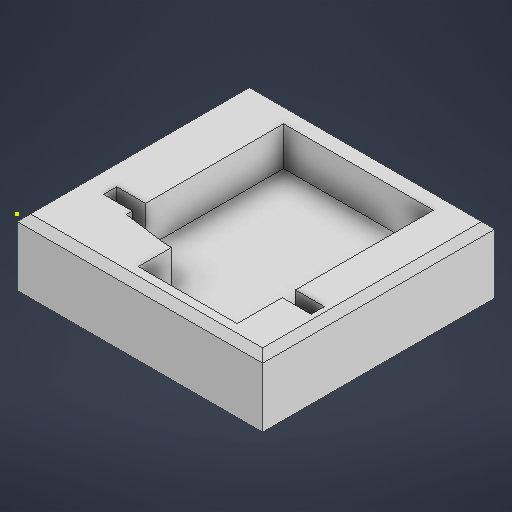
# Autodesk Inventor part: servo_sandbox
Saved by Autodesk Inventor 2026.1 (Build 301233020, 233B)
## iProperties
Created: 2026-02-12
Part Number: servo_sandbox
Material: Generic
Document SubType Name: Modeling
Designer: Dylan
Density: 1 g/cm^3
Appearance: Default
Author: Dylan
Autodesk Inventor part; units mm, degrees
ref_plane "YZ Plane" through (0, 0, 0) normal (1, 0, 0) x (0, 1, 0)
ref_plane "XZ Plane" through (0, 0, 0) normal (0, 1, 0) x (-1, 0, 0)
ref_plane "XY Plane" through (0, 0, 0) normal (0, 0, 1) x (1, 0, 0)
sketch "Sketch2" plane through (0, 0, 0) normal (0, 1, 0) x (-1, 0, 0)
  line L0 (0, 0) -> (-37, 0)
  line L1 (-37, 0) -> (-37, -35)
  line L2 (-37, -35) -> (0, -35)
  line L3 (0, -35) -> (0, 0)
  dimension "d4" = 37
  dimension "d5" = 35
  constraints: 8 end point, 2 parallel, 1 horizontal, 1 perpendicular
  measures "d4" distance of L2.end L1.end
  measures "d5" distance of L1.end L0.end
extrude "Extrusion2" add sketch "Sketch2" along normal blind 10
sketch "Sketch3" plane through (0, 10, 0) normal (0, 1, 0) x (1, 0, 0)
  point P0 (0, 0)
sketch "Sketch4" plane through (0, 10, 0) normal (0, 1, 0) x (1, 0, 0)
  line L0 (30.9066, 2.247) -> (16.0066, 2.247)
  line L1 (16.0066, 2.247) -> (16.0066, 7.247)
  line L2 (16.0066, 7.247) -> (15.0066, 7.247)
  line L3 (30.9066, 2.247) -> (30.9066, 9.047)
  line L4 (30.9066, 9.047) -> (35.2566, 9.047)
  line L5 (35.2566, 9.047) -> (35.2566, 11.047)
  line L6 (35.2566, 11.047) -> (30.9066, 11.047)
  line L7 (30.9066, 11.047) -> (30.9066, 31.847)
  line L8 (30.9066, 31.847) -> (8.3066, 31.847)
  line L9 (8.3066, 31.847) -> (8.3066, 11.047)
  line L10 (8.3066, 11.047) -> (3.9566, 11.047)
  line L11 (3.9566, 11.047) -> (3.9566, 9.047)
  line L12 (3.9566, 9.047) -> (8.3066, 9.047)
  line L13 (8.3066, 9.047) -> (8.3066, 8.147)
  line L14 (8.3066, 8.147) -> (15.0066, 7.247)
  point P0 (0, 0)
  dimension "d8" = 14.9
  dimension "d9" = 5
  dimension "d10" = 1
  dimension "d11" = 6.8
  dimension "d12" = 4.35
  dimension "d13" = 2
  dimension "d14" = 20.8
  dimension "d15" = 22.6
  dimension "d16" = 4.35
  dimension "d17" = 0.9
  constraints: 30 end point, 9 perpendicular, 4 point on line, 2 horizontal, 1 vertical
  measures "d8" distance of L0.start L0.end
  measures "d9" distance of L0.end L1.end
  measures "d10" distance of L1.end L2.end
  measures "d11" distance of L0.start L3.end
  measures "d12" distance of L3.end L4.end
  measures "d13" distance of L4.end L5.end
  measures "d14" distance of L6.end L7.end
  measures "d15" distance of L7.end L8.end
  measures "d16" distance of L9.end L10.end
  measures "d17" distance of L12.end L13.end
extrude "Extrusion3" cut sketch "Sketch4" against normal blind 5.85
chamfer "Chamfer1" distance 1 angle 45 4 edges at (37, 10, -17.5) (18.5, 10, -35) (0, 10, -17.5) (18.5, 10, 0)
body "Solid2"
